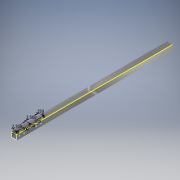
# Autodesk Inventor part: 15102898-16-P-0216
Saved by Autodesk Inventor 2017 (Build 210142000, 142)
## iProperties
Created: 2016-10-06
Part Number: 15102898-16-P-0216
Material: Aluminum 6061
Document SubType Name: Modeling
Designer: gus
Density: 2.7 g/cm^3
Appearance: Aluminum - Flat
Mass: 558.645 g
Surface Area: 1315.32 cm^2
Volume: 206.905 cm^3
Author: gus
Autodesk Inventor part; units mm, degrees
ref_plane "YZ Plane" through (0, 0, 0) normal (1, 0, 0) x (0, 1, 0)
ref_plane "XZ Plane" through (0, 0, 0) normal (0, 1, 0) x (-1, 0, 0)
ref_plane "XY Plane" through (0, 0, 0) normal (0, 0, 1) x (1, 0, 0)
sketch "Sketch1" plane through (0, 0, 0) normal (0, 0, 1) x (1, 0, 0)
  line L0 (0, 0) -> (-25.4, 0)
  line L1 (-25.4, 0) -> (-25.4, 25.4)
  line L2 (-25.4, 25.4) -> (0, 25.4)
  line L3 (0, 25.4) -> (0, 0)
  line L4 (-22.225, 22.225) -> (-22.225, 3.175)
  line L5 (-22.225, 3.175) -> (-3.175, 3.175)
  line L6 (-3.175, 3.175) -> (-3.175, 22.225)
  line L7 (-3.175, 22.225) -> (-22.225, 22.225)
  dimension "d0" = 25.4
  dimension "d1" = 25.4
  dimension "d2" = 3.175
  constraints: 16 end point, 4 parallel, 2 perpendicular, 1 horizontal, 3 other
  measures "d0" distance of L1.end L2.end
  measures "d1" distance of L0.end L1.end
  measures "d2" distance between parallel lines of L1 L4
extrude "Extrusion1" add sketch "Sketch1" along normal blind 736.6
sketch "Sketch2" plane through (-25.4, 25.4, 0) normal (0, 1, 0) x (1, 0, 0)
  circle A0 centre (12.7, -177.8) radius 3.175
  line L0 (0, 0) -> (0, -736.6) projected
  line L1 (0, 0) -> (25.4, 0) projected
  dimension "d5" = 6.35
  dimension "d6" = 12.7
  dimension "d7" = 177.8
  constraints: 1 centre point
  measures "d5" diameter of A0
  measures "d6" distance from line of L0 A0.centre
  measures "d7" distance from line of L1 A0.centre
extrude "Extrusion2" cut sketch "Sketch2" against normal blind 25.4
sketch "Sketch3" plane through (-25.4, 0, 0) normal (-1, 0, 0) x (0, 0, 1)
  circle A0 centre (723.9, 12.7) radius 3.175
  line L0 (0, 0) -> (736.6, 0) projected
  line L1 (736.6, 25.4) -> (736.6, 0) projected
  line L2 (736.6, 12.7) -> (584.2, 12.7) construction
  circle A1 centre (701.675, 12.7) radius 3.175
  circle A2 centre (644.525, 12.7) radius 3.175
  circle A3 centre (622.3, 12.7) radius 3.175
  dimension "d10" = 6.35
  dimension "d11" = 12.7
  dimension "d12" = 152.4
  dimension "d13" = 12.7
  dimension "d14" = 12.7
  dimension "d15" = 6.35
  dimension "d16" = 22.225
  dimension "d17" = 6.35
  dimension "d18" = 6.35
  dimension "d19" = 57.15
  dimension "d20" = 22.225
  constraints: 4 centre point, 3 point on line, 2 end point, 1 horizontal, 1 midpoint
  measures "d10" diameter of A0
  measures "d11" distance from line of L0 A0.centre
  measures "d12" distance of L2.start L2.end
  measures "d13" distance between parallel lines of L0 L2
  measures "d14" distance from line of L1 A0.centre
  measures "d15" diameter of A1
  measures "d16" distance of A0.centre A1.centre
  measures "d17" diameter of A2
  measures "d18" diameter of A3
  measures "d19" distance of A1.centre A2.centre
  measures "d20" distance of A3.centre A2.centre
extrude "Extrusion3" cut sketch "Sketch3" against normal blind 25.4
sketch "Sketch4" plane through (-25.4, 25.4, 0) normal (0, 1, 0) x (1, 0, 0)
  circle A0 centre (12.7, -723.9) radius 3.175
  circle A1 centre (12.7, -660.4) radius 3.175
  circle A2 centre (12.7, -596.9) radius 3.175
  line L0 (25.4, 0) -> (25.4, -736.6) projected
  line L1 (25.4, -736.6) -> (0, -736.6) projected
  circle A3 centre (12.7, -12.7) radius 3.175
  circle A4 centre (12.7, -92.075) radius 3.175
  line L2 (0, 0) -> (25.4, 0) projected
  line L3 (20.6375, -584.2) -> (4.7625, -575.0346)
  line L4 (4.7625, -575.0346) -> (20.6375, -565.8691)
  line L5 (20.6375, -565.8691) -> (20.6375, -584.2)
  line L6 (22.225, 0) -> (22.225, -736.6) projected
  line L7 (0, 0) -> (0, -736.6) projected
  line L8 (4.7625, -570.2721) -> (20.6375, -561.1066)
  line L9 (20.6375, -561.1066) -> (4.7625, -551.9412)
  line L10 (4.7625, -551.9412) -> (4.7625, -570.2721)
  line L11 (20.6375, -533.1666) -> (4.7625, -524.0012)
  line L12 (4.7625, -542.3321) -> (20.6375, -533.1666)
  line L13 (4.7625, -524.0012) -> (4.7625, -542.3321)
  line L14 (4.7625, -547.0946) -> (20.6375, -537.9291)
  line L15 (20.6375, -556.26) -> (4.7625, -547.0946)
  line L16 (20.6375, -537.9291) -> (20.6375, -556.26)
  line L17 (20.6375, -505.2266) -> (4.7625, -496.0612)
  line L18 (4.7625, -514.3921) -> (20.6375, -505.2266)
  line L19 (4.7625, -496.0612) -> (4.7625, -514.3921)
  line L20 (4.7625, -519.1546) -> (20.6375, -509.9891)
  line L21 (20.6375, -528.32) -> (4.7625, -519.1546)
  line L22 (20.6375, -509.9891) -> (20.6375, -528.32)
  line L23 (20.6375, -477.2866) -> (4.7625, -468.1212)
  line L24 (4.7625, -486.4521) -> (20.6375, -477.2866)
  line L25 (4.7625, -468.1212) -> (4.7625, -486.4521)
  line L26 (4.7625, -491.2146) -> (20.6375, -482.0491)
  line L27 (20.6375, -500.38) -> (4.7625, -491.2146)
  line L28 (20.6375, -482.0491) -> (20.6375, -500.38)
  line L29 (20.6375, -449.3466) -> (4.7625, -440.1812)
  line L30 (4.7625, -458.5121) -> (20.6375, -449.3466)
  line L31 (4.7625, -440.1812) -> (4.7625, -458.5121)
  line L32 (4.7625, -463.2746) -> (20.6375, -454.1091)
  line L33 (20.6375, -472.44) -> (4.7625, -463.2746)
  line L34 (20.6375, -454.1091) -> (20.6375, -472.44)
  line L35 (20.6375, -421.4066) -> (4.7625, -412.2412)
  line L36 (4.7625, -430.5721) -> (20.6375, -421.4066)
  line L37 (4.7625, -412.2412) -> (4.7625, -430.5721)
  line L38 (4.7625, -435.3346) -> (20.6375, -426.1691)
  line L39 (20.6375, -444.5) -> (4.7625, -435.3346)
  line L40 (20.6375, -426.1691) -> (20.6375, -444.5)
  line L41 (20.6375, -393.4666) -> (4.7625, -384.3012)
  line L42 (4.7625, -402.6321) -> (20.6375, -393.4666)
  line L43 (4.7625, -384.3012) -> (4.7625, -402.6321)
  line L44 (4.7625, -407.3946) -> (20.6375, -398.2291)
  line L45 (20.6375, -416.56) -> (4.7625, -407.3946)
  line L46 (20.6375, -398.2291) -> (20.6375, -416.56)
  line L47 (20.6375, -365.5266) -> (4.7625, -356.3612)
  line L48 (4.7625, -374.6921) -> (20.6375, -365.5266)
  line L49 (4.7625, -356.3612) -> (4.7625, -374.6921)
  line L50 (4.7625, -379.4546) -> (20.6375, -370.2891)
  line L51 (20.6375, -388.62) -> (4.7625, -379.4546)
  line L52 (20.6375, -370.2891) -> (20.6375, -388.62)
  line L53 (20.6375, -337.5866) -> (4.7625, -328.4212)
  line L54 (4.7625, -346.7521) -> (20.6375, -337.5866)
  line L55 (4.7625, -328.4212) -> (4.7625, -346.7521)
  line L56 (4.7625, -351.5146) -> (20.6375, -342.3491)
  line L57 (20.6375, -360.68) -> (4.7625, -351.5146)
  line L58 (20.6375, -342.3491) -> (20.6375, -360.68)
  line L59 (20.6375, -309.6466) -> (4.7625, -300.4812)
  line L60 (4.7625, -318.8121) -> (20.6375, -309.6466)
  line L61 (4.7625, -300.4812) -> (4.7625, -318.8121)
  line L62 (4.7625, -323.5746) -> (20.6375, -314.4091)
  line L63 (20.6375, -332.74) -> (4.7625, -323.5746)
  line L64 (20.6375, -314.4091) -> (20.6375, -332.74)
  line L65 (20.6375, -281.7066) -> (4.7625, -272.5412)
  line L66 (4.7625, -290.8721) -> (20.6375, -281.7066)
  line L67 (4.7625, -272.5412) -> (4.7625, -290.8721)
  line L68 (4.7625, -295.6346) -> (20.6375, -286.4691)
  line L69 (20.6375, -304.8) -> (4.7625, -295.6346)
  line L70 (20.6375, -286.4691) -> (20.6375, -304.8)
  line L71 (20.6375, -253.7666) -> (4.7625, -244.6012)
  line L72 (4.7625, -262.9321) -> (20.6375, -253.7666)
  line L73 (4.7625, -244.6012) -> (4.7625, -262.9321)
  line L74 (4.7625, -267.6946) -> (20.6375, -258.5291)
  line L75 (20.6375, -276.86) -> (4.7625, -267.6946)
  line L76 (20.6375, -258.5291) -> (20.6375, -276.86)
  line L77 (20.6375, -225.8266) -> (4.7625, -216.6612)
  line L78 (4.7625, -234.9921) -> (20.6375, -225.8266)
  line L79 (4.7625, -216.6612) -> (4.7625, -234.9921)
  line L80 (4.7625, -239.7546) -> (20.6375, -230.5891)
  line L81 (20.6375, -248.92) -> (4.7625, -239.7546)
  line L82 (20.6375, -230.5891) -> (20.6375, -248.92)
  line L83 (20.6375, -197.8866) -> (4.7625, -188.7212)
  line L84 (4.7625, -207.0521) -> (20.6375, -197.8866)
  line L85 (4.7625, -188.7212) -> (4.7625, -207.0521)
  line L86 (4.7625, -211.8146) -> (20.6375, -202.6491)
  line L87 (20.6375, -220.98) -> (4.7625, -211.8146)
  line L88 (20.6375, -202.6491) -> (20.6375, -220.98)
  line L89 (20.6375, -169.9466) -> (4.7625, -160.7812)
  line L90 (4.7625, -179.1121) -> (20.6375, -169.9466)
  line L91 (4.7625, -160.7812) -> (4.7625, -179.1121)
  line L92 (4.7625, -183.8746) -> (20.6375, -174.7091)
  line L93 (20.6375, -193.04) -> (4.7625, -183.8746)
  line L94 (20.6375, -174.7091) -> (20.6375, -193.04)
  line L95 (20.6375, -142.0066) -> (4.7625, -132.8412)
  line L96 (4.7625, -151.1721) -> (20.6375, -142.0066)
  line L97 (4.7625, -132.8412) -> (4.7625, -151.1721)
  line L98 (4.7625, -155.9346) -> (20.6375, -146.7691)
  line L99 (20.6375, -165.1) -> (4.7625, -155.9346)
  line L100 (20.6375, -146.7691) -> (20.6375, -165.1)
  dimension "d23" = 63.5
  dimension "d24" = 63.5
  dimension "d25" = 6.35
  dimension "d26" = 12.7
  dimension "d27" = 12.7
  dimension "d28" = 12.7
  dimension "d29" = 12.7
  dimension "d32" = 6.35
  dimension "d33" = 6.35
  dimension "d34" = 12.7
  dimension "d35" = 92.075
  dimension "d36" = 12.7
  dimension "d37" = 12.7
  dimension "d38" = 4.7625
  dimension "d39" = 1.5875
  dimension "d40" = 152.4
  dimension "d41" = 4.7625
  dimension "d42" = 4.7625
  dimension "d45" = 27.94
  constraints: 208 end point, 5 centre point, 5 equal length, 2 equal radius, 2 vertical, 1 parallel, 180 other
  measures "d23" distance of A1.centre A2.centre
  measures "d24" distance of A0.centre A1.centre
  measures "d25" diameter of A2
  measures "d26" distance from line of L0 A2.centre
  measures "d27" distance from line of L0 A1.centre
  measures "d28" distance from line of L0 A0.centre
  measures "d29" distance from line of L1 A0.centre
  measures "d32" diameter of A3
  measures "d33" diameter of A4
  measures "d34" distance from line of L2 A3.centre
  measures "d35" distance from line of L2 A4.centre
  measures "d36" distance from line of L0 A4.centre
  measures "d37" distance from line of L0 A3.centre
  measures "d38" distance from line of L7 L3.end
  measures "d39" distance between parallel lines of L6 L5
  measures "d40" distance from line of L1 L3.start
  measures "d41" distance between parallel lines of L7 L10
  measures "d42" distance of L4.end L8.end
  measures "d45" distance of L8.end L11.start
extrude "Extrusion4" cut sketch "Sketch4" against normal blind 25.4 contours A0 | A1 | A2 | A3 | A4 | L3 L4 L5 | L10 L9 L8 | L12 L13 L11 | L18 L19 L17 | L20 L22 L21 | L24 L25 L23 | L26 L28 L27 | L30 L31 L29 | L32 L34 L33 | L36 L37 L35 | L38 L40 L39
extrude "Extrusion5" cut sketch "Sketch4" against normal blind 25.4 contours L14 L16 L15 | L42 L43 L41 | L44 L46 L45 | L48 L49 L47 | L50 L52 L51 | L54 L55 L53 | L56 L58 L57 | L60 L61 L59 | L62 L64 L63 | L66 L67 L65 | L68 L70 L69 | L72 L73 L71 | L74 L76 L75 | L78 L79 L77 | L80 L82 L81 | L84 L85 L83 | L86 L88 L87 | L90 L91 L89 | L92 L94 L93 | L96 L97 L95 | L98 L100 L99
body "Solid1"
